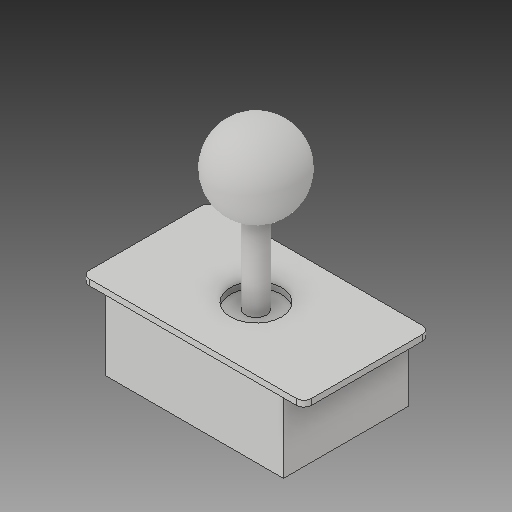
# Autodesk Inventor part: Joy_Stick
Saved by Autodesk Inventor 2017 (Build 210142000, 142)
## iProperties
Created: 2019-03-30
Part Number: Joy_Stick
Material: Generic
Document SubType Name: Modeling
Designer: Mitch
Density: 1 g/cm^3
Appearance: Default
Mass: 160.596 g
Surface Area: 237.729 cm^2
Volume: 160.596 cm^3
Author: Mitch
Autodesk Inventor part; units mm, degrees
ref_plane "YZ Plane" through (0, 0, 0) normal (1, 0, 0) x (0, 1, 0)
ref_plane "XZ Plane" through (0, 0, 0) normal (0, 1, 0) x (-1, 0, 0)
ref_plane "XY Plane" through (0, 0, 0) normal (0, 0, 1) x (1, 0, 0)
sketch "Sketch1" plane through (0, 0, 0) normal (0, 1, 0) x (-1, 0, 0)
  line L0 (0, 0) -> (95, 0)
  line L1 (95, 0) -> (95, -54)
  line L2 (95, -54) -> (0, -54)
  line L3 (0, -54) -> (0, 0)
  dimension "d0" = 95
  dimension "d1" = 54
  constraints: 8 end point, 2 parallel, 1 horizontal, 1 perpendicular
  measures "d0" distance of L1.end L2.end
  measures "d1" distance of L0.end L1.end
extrude "Extrusion1" add sketch "Sketch1" along normal blind 2.54
fillet "Fillet1" radius 3.175 4 edges at (0, 1.27, 0) (-95, 1.27, 0) (0, 1.27, -54) (-95, 1.27, -54)
sketch "Sketch2" plane through (0, 0, 0) normal (0, -1, 0) x (1, 0, 0)
  arc A0 (-95, -50.825) -> (-91.825, -54) centre (-91.825, -50.825) ccw projected
  line L0 (-91.825, -54) -> (-3.175, -54) projected
  arc A1 (-3.175, -54) -> (0, -50.825) centre (-3.175, -50.825) ccw projected
  line L1 (0, -50.825) -> (0, -3.175) projected
  arc A2 (0, -3.175) -> (-3.175, 0) centre (-3.175, -3.175) ccw projected
  line L2 (-3.175, 0) -> (-91.825, 0) projected
  arc A3 (-91.825, 0) -> (-95, -3.175) centre (-91.825, -3.175) ccw projected
  line L3 (-95, -3.175) -> (-95, -50.825) projected
  line L4 (-85.602, -54) -> (-9.402, -54)
  line L5 (-9.402, -54) -> (-9.402, -0.66)
  line L6 (-9.402, -0.66) -> (-85.602, -0.66)
  line L7 (-85.602, -0.66) -> (-85.602, -54)
  point P0 (0, 0)
  dimension "d5" = 76.2
  dimension "d6" = 53.34
  dimension "d7" = 0
  dimension "d8" = 9.398
  constraints: 8 end point, 2 parallel, 1 horizontal, 1 perpendicular
  measures "d5" distance of L6.end L5.end
  measures "d6" distance of L5.end L4.end
  measures "d7" distance between parallel lines of L4 L0
  measures "d8" distance between parallel lines of L3 L7
extrude "Extrusion2" add sketch "Sketch2" along normal blind 30.48 contours L7 L6 L5 L0
sketch "Sketch3" plane through (0, 2.54, 0) normal (0, 1, 0) x (1, 0, 0)
  arc A0 (-91.825, 54) -> (-95, 50.825) centre (-91.825, 50.825) ccw projected
  arc A1 (-91.825, 54) -> (-95, 50.825) centre (-91.825, 50.825) ccw projected
  line L0 (-95, 50.825) -> (-95, 3.175) projected
  arc A2 (-95, 3.175) -> (-91.825, 0) centre (-91.825, 3.175) ccw projected
  line L1 (-91.825, 0) -> (-3.175, 0) projected
  arc A3 (-3.175, 0) -> (0, 3.175) centre (-3.175, 3.175) ccw projected
  line L2 (0, 3.175) -> (0, 50.825) projected
  arc A4 (0, 50.825) -> (-3.175, 54) centre (-3.175, 50.825) ccw projected
  line L3 (-3.175, 54) -> (-91.825, 54) projected
  line L4 (-3.175, 3.175) -> (-91.825, 50.825)
  circle A5 centre (-47.5, 27) radius 10.922
  point P0 (0, 0)
  dimension "d11" = 21.844
  constraints: 2 end point, 1 centre point, 1 midpoint
  measures "d11" diameter of A5
extrude "Extrusion3" cut sketch "Sketch3" against normal blind 2.54 contours A5 L4 | L4 A5
sketch "Sketch4" plane through (-47.5, 0, -27) normal (0, 1, 0) x (1, 0, 0)
  circle A0 centre (0, 0) radius 4.4704
  point P0 (47.5, -27)
  dimension "d14" = 8.9408
  constraints: 1 centre point
  measures "d14" diameter of A0
extrude "Extrusion4" add sketch "Sketch4" along normal blind 43.815
ref_plane "Work Plane1" through (-47.5, 52.315, -27) normal (0, 1, 0) x (1, 0, 0)
sketch "Sketch5" plane through (-47.5, 52.315, -27) normal (0, 1, 0) x (1, 0, 0)
  arc A0 (-17.5, 0) -> (17.5, 0) centre (0, 0) ccw
  line L0 (17.5, 0) -> (-17.5, 0)
  point P0 (47.5, -27)
  dimension "d18" = 35
  constraints: 2 end point, 2 point on circle, 1 centre point, 1 horizontal
  measures "d18" diameter of A0
revolve "Revolution1" add sketch "Sketch5" angle 360 about axis through (-30, 52.315, -27) along (-1, 0, 0)
body "Solid1"
